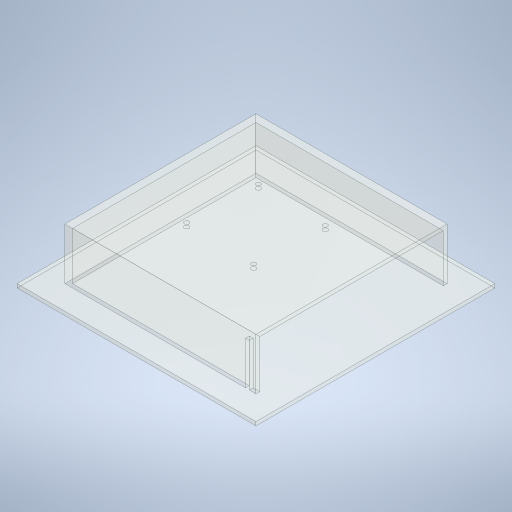
# Autodesk Inventor part: Acrylic Casing
Saved by Autodesk Inventor 2024 (Build 280153000, 153)
## iProperties
Created: 2023-07-17
Part Number: Acrylic Casing
Material: Acetal Resin, White
Document SubType Name: Modeling
Designer: javie
Density: 1.425 g/cm^3
Appearance: Clear
Author: javie
Autodesk Inventor part; units mm, degrees
ref_plane "YZ Plane" through (0, 0, 0) normal (1, 0, 0) x (0, 1, 0)
ref_plane "XZ Plane" through (0, 0, 0) normal (0, 1, 0) x (-1, 0, 0)
ref_plane "XY Plane" through (0, 0, 0) normal (0, 0, 1) x (1, 0, 0)
sketch "Sketch1" plane through (0, 0, 0) normal (0, 1, 0) x (-1, 0, 0)
  line L0 (-125, -125) -> (125, -125)
  line L1 (125, -125) -> (125, 125)
  line L2 (125, 125) -> (-125, 125)
  line L3 (-125, 125) -> (-125, -125)
  line L4 (-125, -125) -> (125, 125) construction
  line L5 (125, -125) -> (-125, 125) construction
  point P0 (0, 0)
  dimension "Width" = 250
  dimension "Length" = 250
  constraints: 12 end point, 2 midpoint, 2 parallel, 1 horizontal, 1 perpendicular
  measures "Width" distance of L2.end L1.end
  measures "Length" distance of L1.end L0.end
extrude "Main Body Extrusion" add sketch "Sketch1" along normal blind 4
sketch "Sketch3" plane through (0, 4, 0) normal (0, 1, 0) x (1, 0, 0)
  line L0 (96, -96) -> (-96, -96)
  line L1 (-96, -96) -> (-96, 96)
  line L2 (-96, 96) -> (96, 96)
  line L3 (96, -96) -> (-96, 96) construction
  line L4 (-96, -96) -> (96, 96) construction
  line L5 (-125, 125) -> (-125, -125) projected
  line L6 (125, -125) -> (125, 125) projected
  line L7 (-125, -125) -> (125, -125) projected
  line L8 (100, -100) -> (-100, -100)
  line L9 (-100, -100) -> (-100, 100)
  line L10 (-100, 100) -> (100, 100)
  line L11 (100, -100) -> (-100, 100) construction
  line L12 (-100, -100) -> (100, 100) construction
  line L13 (96, 96) -> (100, 96)
  line L14 (96, -96) -> (100, -96)
  line L15 (100, 100) -> (100, 96)
  line L16 (100, -96) -> (100, -100)
  point P0 (0, 0)
  dimension "d16" = 192
  dimension "d17" = 200
  dimension "d18" = 200
  constraints: 28 end point, 7 perpendicular, 4 midpoint, 4 parallel, 2 horizontal
  measures "d16" distance of L0.end L1.end
  measures "d17" distance of L9.end L10.end
  measures "d18" distance of L8.end L9.end
extrude "Extrusion3" add sketch "Sketch3" along normal blind 50 from surface at 0
sketch "Sketch8" plane through (0, 4, 0) normal (0, 1, 0) x (1, 0, 0)
  line L0 (100, 100) -> (100, 96) projected
  line L1 (-96, 96) -> (-96, -96) projected
  line L2 (100, 96) -> (-96, 96) projected
  line L3 (-125, -125) -> (125, -125) projected
  line L4 (89, 96) -> (93, 96)
  line L5 (93, 96) -> (93, -125)
  line L6 (93, -125) -> (89, -125)
  line L7 (89, -125) -> (89, 96)
  line L8 (89, -96) -> (85, -96)
  line L9 (85, -96) -> (85, 96)
  line L10 (85, 96) -> (89, 96)
  line L11 (89, 96) -> (89, -96)
  line L12 (93, 96) -> (97, 96)
  line L13 (97, 96) -> (97, -96)
  line L14 (97, -96) -> (93, -96)
  line L15 (93, -96) -> (93, 96)
  point P0 (0, 0)
  point P1 (89, -125)
  dimension "d39" = 4
  dimension "d40" = 185
  dimension "d47" = 4
  dimension "d48" = 4
  constraints: 24 end point, 6 parallel, 5 point on line, 3 horizontal, 3 perpendicular
  measures "d39" distance of L5.end L6.end
  measures "d40" distance between parallel lines of L1 L7
  measures "d47" distance of L9.end L10.end
  measures "d48" distance of L13.end L14.end
extrude "Extrusion8" cut sketch "Sketch8" along normal blind 2 contours L13 L14 L5 L2 | L7 L8 L9 L2
sketch "Sketch9" plane through (-100, 54, 100) normal (0, 0, 1) x (1, 0, 0)
  line L0 (0, -50) -> (200, -50) projected
  line L1 (193.0019, -50) -> (189.0019, -50)
  line L2 (189.0019, -50) -> (189.0019, -5)
  line L3 (189.0019, -5) -> (193.0019, -5)
  line L4 (193.0019, -5) -> (193.0019, -50)
  point P0 (100, -54)
  dimension "d41" = 4
  dimension "d42" = 45
  constraints: 8 end point, 2 parallel, 1 horizontal, 1 perpendicular, 1 point on line
  measures "d41" distance of L2.end L3.end
  measures "d42" distance of L1.end L2.end
extrude "Extrusion9" cut sketch "Sketch9" against normal up to surface (4 mm away)
sketch "Sketch10" plane through (-100, 54, -100) normal (0, 1, 0) x (1, 0, 0)
  line L0 (0, -200) -> (0, 0) projected
  line L1 (200, 0) -> (200, -4) projected
  line L2 (0, -200) -> (200, -200)
  line L3 (200, -200) -> (200, 0)
  line L4 (200, 0) -> (0, 0)
  line L5 (0, 0) -> (0, -200)
  point P0 (100, -100)
  constraints: 8 end point, 2 parallel, 1 horizontal, 1 perpendicular
extrude "Extrusion10" add sketch "Sketch10" along normal blind 4
sketch "Sketch11" plane through (-100, 58, -100) normal (0, 1, 0) x (1, 0, 0)
  line L0 (50, -150) -> (150, -150)
  line L1 (150, -150) -> (150, -50)
  line L2 (150, -50) -> (50, -50)
  line L3 (50, -50) -> (50, -150)
  line L4 (50, -150) -> (150, -50) construction
  line L5 (150, -150) -> (50, -50) construction
  point P0 (100, -100)
  point P1 (65, -62.5)
  point P2 (62.5, -135)
  point P3 (135, -137.5)
  point P4 (137.5, -65)
  dimension "d56" = 100
  dimension "d57" = 100
  dimension "d58" = 12.5
  dimension "d59" = 15
  dimension "d62" = 360
  constraints: 12 end point, 2 midpoint, 2 parallel, 1 horizontal, 1 perpendicular, 5 other
  measures "d56" distance of L2.end L1.end
  measures "d57" distance of L1.end L0.end
  measures "d58" distance from line of L2 point (65, -62.5)
  measures "d59" distance from line of L3 point (65, -62.5)
hole "Hole1" at (-35, 58, -37.5) at (37.5, 58, -35) at (35, 58, 37.5) at (-37.5, 58, 35) direction (0, -1, 0) diameter 5 depth 4
body "Solid1"
